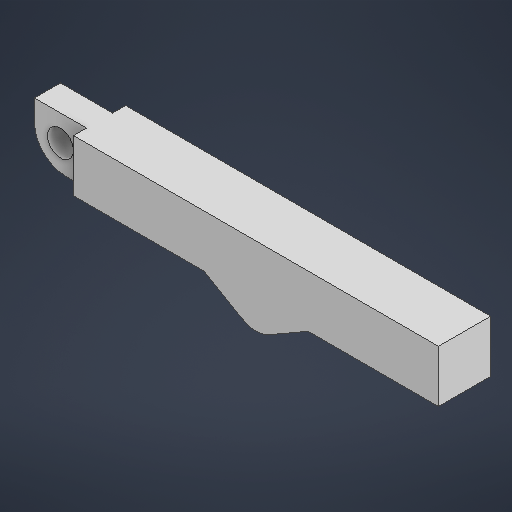
# Autodesk Inventor part: Press_Upper_Arm
Saved by Autodesk Inventor 2026.1 (Build 301233020, 233B)
## iProperties
Created: 2025-10-06
Part Number: Press_Upper_Arm
Material: Generic
Document SubType Name: Modeling
Designer: Gamec
Density: 1 g/cm^3
Appearance: Default
Author: Gamec
Autodesk Inventor part; units mm, degrees
ref_plane "YZ Plane" through (0, 0, 0) normal (1, 0, 0) x (0, 1, 0)
ref_plane "XZ Plane" through (0, 0, 0) normal (0, 1, 0) x (-1, 0, 0)
ref_plane "XY Plane" through (0, 0, 0) normal (0, 0, 1) x (1, 0, 0)
sketch "Sketch1" plane through (0, 0, 0) normal (0, 0, 1) x (1, 0, 0)
  line L0 (-50.8, -6.35) -> (50.8, -6.35)
  line L1 (50.8, -6.35) -> (50.8, 6.35)
  line L2 (50.8, 6.35) -> (-50.8, 6.35)
  line L3 (-50.8, 6.35) -> (-50.8, -6.35)
  line L4 (-50.8, -6.35) -> (50.8, 6.35) construction
  line L5 (50.8, -6.35) -> (-50.8, 6.35) construction
  point P0 (0, 0)
  dimension "d0" = 101.6
  dimension "d1" = 12.7
  constraints: 12 end point, 2 midpoint, 2 parallel, 1 horizontal, 1 perpendicular
  measures "d0" distance of L2.end L1.end
  measures "d1" distance of L1.end L0.end
extrude "Extrusion1" add sketch "Sketch1" along normal blind 12.7
fillet "Fillet1" radius 7.62 1 edges at (-50.8, -6.35, 6.35)
sketch "Sketch2" plane through (0, 0, 12.7) normal (0, 0, 1) x (1, 0, 0)
  circle A0 centre (-44.45, 0) radius 3.175
  line L0 (-50.8, 6.35) -> (-50.8, 1.27) projected
  line L1 (50.8, 6.35) -> (-50.8, 6.35) projected
  point P0 (0, 0)
  dimension "d5" = 6.35
  dimension "d6" = 6.35
  dimension "d7" = 6.35
  constraints: 1 centre point
  measures "d5" diameter of A0
  measures "d6" distance from line of L0 A0.centre
  measures "d7" distance from line of L1 A0.centre
extrude "Extrusion2" cut sketch "Sketch2" against normal blind 12.7
sketch "Sketch3" plane through (0, 0, 12.7) normal (0, 0, 1) x (1, 0, 0)
  line L0 (-43.18, -6.35) -> (50.8, -6.35) projected
  circle A0 centre (6.35, -6.35) radius 6.35
  line L1 (-6.35, -6.35) -> (3.175, -11.8493)
  line L2 (19.05, -6.35) -> (9.525, -11.8493)
  line L3 (-50.8, 6.35) -> (-50.8, 1.27) projected
  point P0 (0, 0)
  dimension "d10" = 12.7
  dimension "d11" = 12.7
  dimension "d12" = 12.7
  dimension "d15" = 57.15
  constraints: 4 end point, 3 point on line, 2 point on circle, 2 tangent, 1 centre point
  measures "d10" diameter of A0
  measures "d11" distance of A0.centre L1.start
  measures "d12" distance of A0.centre L2.start
  measures "d15" distance from line of L3 A0.centre
extrude "Extrusion3" add sketch "Sketch3" against normal blind 12.7 contours A0 L0 | L0 L2 A0 | A0 L1 L0 picked at (4.9799, -8.3631)
sketch "Sketch4" plane through (-50.8, 6.35, 0) normal (0, 1, 0) x (1, 0, 0)
  line L0 (7.62, -12.7) -> (0, -12.7) projected
  line L1 (0, -12.7) -> (12.7, -12.7)
  line L2 (12.7, -12.7) -> (12.7, -9.525)
  line L3 (12.7, -9.525) -> (0, -9.525)
  line L4 (0, -9.525) -> (0, -12.7)
  line L5 (0, 0) -> (12.7, 0)
  line L6 (12.7, 0) -> (12.7, -3.175)
  line L7 (12.7, -3.175) -> (0, -3.175)
  line L8 (0, -3.175) -> (0, 0)
  point P0 (50.8, 0)
  dimension "d16" = 12.7
  dimension "d17" = 3.175
  dimension "d18" = 3.175
  constraints: 16 end point, 4 parallel, 2 horizontal, 2 perpendicular, 2 point on line
  measures "d16" distance of L3.end L2.end
  measures "d17" distance of L2.end L1.end
  measures "d18" distance of L5.end L6.end
extrude "Extrusion4" cut sketch "Sketch4" against normal blind 12.7
body "Solid1"
